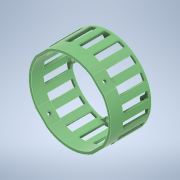
# Autodesk Inventor part: Hoop
Saved by Autodesk Inventor 2022.2 (Build 262287010, 287A)
## iProperties
Created: 2022-02-16
Part Number: Hoop
Material: ABS Plastic
Document SubType Name: Modeling
Designer: smiku
Density: 1.06 g/cm^3
Appearance: Smooth - Dark Forest Green
Author: smiku
Autodesk Inventor part; units mm, degrees
ref_plane "YZ Plane" through (0, 0, 0) normal (1, 0, 0) x (0, 1, 0)
ref_plane "XZ Plane" through (0, 0, 0) normal (0, 1, 0) x (-1, 0, 0)
ref_plane "XY Plane" through (0, 0, 0) normal (0, 0, 1) x (1, 0, 0)
sketch "Sketch1" plane through (0, 0, 0) normal (0, 0, 1) x (1, 0, 0)
  circle A0 centre (0, 0) radius 50
  circle A1 centre (0, 0) radius 47
  circle A2 centre (0, 43) radius 2
  arc A3 (3.5571, 41.1705) -> (-3.5571, 41.1705) centre (0, 43) ccw construction
  arc A4 (-3.5571, 41.1705) -> (-12.8603, 45.2063) centre (-10.6714, 37.5116) ccw
  arc A5 (12.8603, 45.2063) -> (3.5571, 41.1705) centre (10.6714, 37.5116) ccw
  arc A6 (-3.5571, 41.1705) -> (3.5571, 41.1705) centre (0, 43) ccw
  arc A7 (-41.1705, -3.5571) -> (-45.2063, -12.8603) centre (-37.5116, -10.6714) ccw
  arc A8 (-41.1705, -3.5571) -> (-41.1705, 3.5571) centre (-43, 0) ccw
  arc A9 (-45.2063, 12.8603) -> (-41.1705, 3.5571) centre (-37.5116, 10.6714) ccw
  circle A10 centre (-43, 0) radius 2
  arc A11 (3.5571, -41.1705) -> (12.8603, -45.2063) centre (10.6714, -37.5116) ccw
  arc A12 (3.5571, -41.1705) -> (-3.5571, -41.1705) centre (0, -43) ccw
  arc A13 (-12.8603, -45.2063) -> (-3.5571, -41.1705) centre (-10.6714, -37.5116) ccw
  circle A14 centre (0, -43) radius 2
  arc A15 (41.1705, 3.5571) -> (45.2063, 12.8603) centre (37.5116, 10.6714) ccw
  arc A16 (41.1705, 3.5571) -> (41.1705, -3.5571) centre (43, 0) ccw
  arc A17 (45.2063, -12.8603) -> (41.1705, -3.5571) centre (37.5116, -10.6714) ccw
  circle A18 centre (43, 0) radius 2
  point P0 (-12.8603, -45.2063)
  point P1 (12.8603, -45.2063)
  point P2 (45.2063, -12.8603)
  point P3 (45.2063, 12.8603)
  point P4 (-45.2063, 12.8603)
  point P5 (-45.2063, -12.8603)
  dimension "d0" = 100
  dimension "d4" = 3
  dimension "d19" = 4
  dimension "d20" = 8
  dimension "d22" = 8
  dimension "d25" = 360
  dimension "d27" = 43
  constraints: 28 point on circle, 19 centre point, 5 coincident, 5 tangent, 1 equal radius, 1 vertical alignment, 49 other
  measures "d0" diameter of A0
  measures "d4" radial gap between concentric circles of A0 A1
  measures "d19" diameter of A2
  measures "d20" diameter of A3
  measures "d22" radius of A4
  measures "d27" distance of A2.centre A0.centre
extrude "Extrusion1" add sketch "Sketch1" along normal blind 34 contours A0
sketch "Sketch2" plane through (0, 0, 34) normal (0, 0, -1) x (-1, 0, 0)
  circle A0 centre (0, 0) radius 50 projected
  circle A1 centre (0, 0) radius 47 projected
  line L0 (25.7078, 39.346) -> (39.346, 25.7078) construction
  circle A2 centre (0, 0) radius 47 construction
  line L1 (0, 0) -> (32.5269, 32.5269) construction
  line L2 (0, 0) -> (47, 0) construction
  circle A3 centre (0, 0) radius 50 construction
  line L3 (25.7078, 39.346) -> (39.346, 25.7078)
  line L4 (39.346, 25.7078) -> (41.5106, 27.8724)
  line L5 (41.5106, 27.8724) -> (27.8724, 41.5106)
  line L6 (27.8724, 41.5106) -> (25.7078, 39.346)
  line L7 (-27.8724, 41.5106) -> (-41.5106, 27.8724)
  line L8 (-41.5106, 27.8724) -> (-39.346, 25.7078)
  line L9 (-25.7078, 39.346) -> (-27.8724, 41.5106)
  line L10 (-39.346, 25.7078) -> (-25.7078, 39.346)
  line L11 (-41.5106, -27.8724) -> (-27.8724, -41.5106)
  line L12 (-27.8724, -41.5106) -> (-25.7078, -39.346)
  line L13 (-39.346, -25.7078) -> (-41.5106, -27.8724)
  line L14 (-25.7078, -39.346) -> (-39.346, -25.7078)
  line L15 (27.8724, -41.5106) -> (41.5106, -27.8724)
  line L16 (41.5106, -27.8724) -> (39.346, -25.7078)
  line L17 (25.7078, -39.346) -> (27.8724, -41.5106)
  line L18 (39.346, -25.7078) -> (25.7078, -39.346)
  dimension "d5" = 45
  dimension "d6" = 46
  dimension "d9" = 360
  constraints: 38 end point, 3 equal length, 3 point on circle, 1 horizontal, 1 midpoint, 1 perpendicular, 35 other
  measures "d5" angle of L2 L1
  measures "d6" distance of L1.start L1.end
extrude "Extrusion2" add sketch "Sketch2" against normal blind 15 contours A0 L16 A1 L4 | L4 A1 L6 L5 | L15 L17 A1 L16 | L6 A1 L9 A0 | L3 A1 | A0 L12 A1 L17 | A1 L18 | L9 A1 L8 L7 | L11 L13 A1 L12 | L8 A1 L13 A0 | L10 A1 | A1 L14
sketch "Sketch3" plane through (27.8724, 41.5106, 34) normal (0.7071068, 0.7071068, 0) x (-0.7071068, 0.7071068, 0)
  line L0 (0, 0) -> (-19.2873, 0) construction
  line L1 (0, 0) -> (0, 15) construction
  line L2 (-19.2873, 15) -> (0, 15) construction
  line L3 (-19.2873, 0) -> (-19.2873, 15) construction
  line L4 (0, 0) -> (-19.2873, 0) construction
  line L5 (0, 0) -> (0, 15) construction
  line L6 (-19.2873, 0) -> (0, 15) construction
  circle A0 centre (-9.6437, 7.5) radius 2
  point P0 (-9.6437, -34)
  dimension "d13" = 4
  constraints: 2 end point, 1 centre point, 1 midpoint
  measures "d13" diameter of A0
extrude "Extrusion3" cut sketch "Sketch3" against normal up to next
pattern_circular "Circular Pattern1" count 4 over 360 about axis through (0, 0, -10) along (0, 0, 1) of "Extrusion3"
extrude "Extrusion4" add sketch "Sketch1" along normal blind 3 contours A1 A17 A16 A15 | A5 A6 A4 A1 | A1 A13 A12 A11 | A9 A8 A7 A1
sketch "Sketch4" plane through (0, 0, 3) normal (0, 0, 1) x (1, 0, 0)
  line L0 (0, 0) -> (0, 50) construction
  circle A0 centre (0, 0) radius 50 projected
  line L1 (0, 0) -> (-4.3578, 49.8097)
  line L2 (0, 0) -> (4.3578, 49.8097)
  arc A1 (4.3578, 49.8097) -> (-4.3578, 49.8097) centre (0, 0) ccw
  arc A2 (27.8724, 41.5106) -> (-27.8724, 41.5106) centre (0, 0) ccw projected
  point P0 (0, 50)
  point P1 (4.3578, 49.8097)
  point P2 (-4.3578, 49.8097)
  dimension "d30" = 10
  constraints: 6 end point, 6 point on circle, 1 centre point, 1 coincident, 1 vertical
  measures "d30" angle of L2 L1
extrude "Extrusion5" cut sketch "Sketch4" along normal up to surface (31 mm away) contours L2 L1 A0 picked at (0, 33.3192)
pattern_circular "Circular Pattern2" count 18 over 360 about axis through (0, 0, -10) along (0, 0, 1) of "Extrusion5"
body "Solid1"
